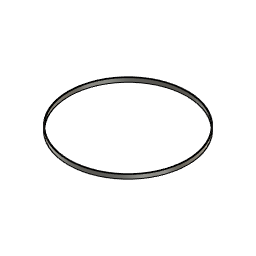
Track Test v2 (Autodesk Fusion 360 design; units mm, degrees)
Autodesk Fusion 360 part; units mm, degrees
note: some values were not read from the file. Set by a fixed rule: which sketch regions a step uses.
sketch "Sketch1" plane through (0, 0, 0) normal (0, 1, 0) x (1, 0, 0)
  line L0 (146.4, -2) -> (146.4, -40)
  line L1 (146.4, -40) -> (144.4, -40)
  line L2 (144.4, -40) -> (144.4, -2)
  line L3 (144.4, -2) -> (146.4, -2)
  dimension "d11" = 2
  dimension "d12" = 38
  constraint perpendicular L0 L1
  constraint perpendicular L1 L2
  constraint perpendicular L0 L3
  measures "d11" distance of L0.end L1.end
  measures "d12" distance of L1.end L2.end
revolve "Revolve1" add sketch "Sketch1" angle 360 about axis through (0, 0, 1.75) along (0, 0, 1)
extrude "Extrude1" cut 1 faces at (140.8818, -35.8449, 40) along direction (0, 0, -1) blind 28
